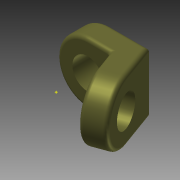
# Autodesk Inventor part: Levier
Saved by Autodesk Inventor 2011 SP2 (Build 150309200, 309)
## iProperties
Created: 2023-03-20
Part Number: Levier
Document SubType Name: Modeling
Designer: utilizator
Density: 1 g/cm^3
Author: utilizator
Autodesk Inventor part; units mm, degrees
ref_plane "YZ Plane" through (0, 0, 0) normal (1, 0, 0) x (0, 1, 0)
ref_plane "XZ Plane" through (0, 0, 0) normal (0, 1, 0) x (-1, 0, 0)
ref_plane "XY Plane" through (0, 0, 0) normal (0, 0, 1) x (1, 0, 0)
sketch "Sketch1" plane through (0, 0, 0) normal (0, 0, 1) x (1, 0, 0)
  line L0 (0, -45.5198) -> (0, 7.5866) projected
  line L1 (-45.6625, 0) -> (21.9753, 0) projected
  line L2 (0, 0) -> (-36, 0)
  line L3 (-36, 0) -> (-36, -12)
  line L4 (-36, -12) -> (-8.4025, -12)
  line L5 (-8.4025, -12) -> (0, 0) construction
  line L6 (0, 0) -> (12.3127, -33.8289)
  line L7 (12.3127, -33.8289) -> (1.0364, -37.9332)
  line L8 (1.0364, -37.9332) -> (-8.4025, -12)
  dimension "d0" = 36
  dimension "d1" = 12
  dimension "d2" = 55
  constraints: 14 end point, 2 perpendicular, 2 symmetric about line, 1 point on line
  measures "d0" distance of L2.start L2.end
  measures "d1" distance of L2.end L3.end
  measures "d2" angle of L5 L2
extrude "Extrusion1" add sketch "Sketch1" along normal blind 32
fillet "Fillet1" radius 16 4 edges at (-36, -6, 32) (6.6746, -35.8811, 32) (6.6746, -35.8811, 0) (-36, -6, 0)
hole "Hole1" at (-20, -12, 16) direction (0, 1, 0) diameter 16 end through all
hole "Hole2" at (-4.4359, -22.8981, 16) direction (0.9396926, 0.3420201, 0) diameter 16 end through all
fillet "Fillet2" radius 2 12 edges at (3.4202, -9.397, 32) (10.7099, -29.4253, 27.3137) (3.4202, -9.397, 0) (-6.4192, -17.4491, 32) (-0.5664, -33.5295, 27.3137) (-6.4192, -17.4491, 0) (-14.2013, -12, 32) (-31.3137, -12, 27.3137) (-14.2013, -12, 0) (-10.0001, 0, 32) (-31.3137, 0, 27.3137) (-10.0001, 0, 0)
fillet "Fillet3" radius 2 3 edges at (-8.4025, -12, 16) (-7.9923, -11.4142, 31.4142) (-7.9923, -11.4142, 0.5858)
body "Solid1"
